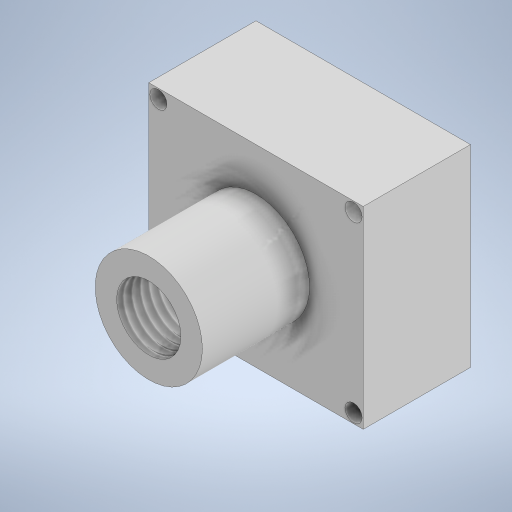
# Autodesk Inventor part: Practica 1 Sofia Lopez
Saved by Autodesk Inventor 2024 (Build 280153000, 153)
## iProperties
Created: 2024-02-06
Part Number: Practica 1 Sofia Lopez
Material: Generic
Document SubType Name: Sheet Metal
Designer: USUARIO
Density: 1 g/cm^3
Sheet Metal Rule: Default
Appearance: Default
Author: USUARIO
Autodesk Inventor part; units mm, degrees
ref_plane "YZ Plane" through (0, 0, 0) normal (1, 0, 0) x (0, 1, 0)
ref_plane "XZ Plane" through (0, 0, 0) normal (0, 1, 0) x (-1, 0, 0)
ref_plane "XY Plane" through (0, 0, 0) normal (0, 0, 1) x (1, 0, 0)
sketch "Sketch1" plane through (0, 0, 0) normal (0, 0, 1) x (1, 0, 0)
  line L0 (-50, 45) -> (50, 45)
  line L1 (50, 45) -> (50, -45)
  line L2 (50, -45) -> (-50, -45)
  line L3 (-50, -45) -> (-50, 45)
  line L4 (-50, 45) -> (50, -45) construction
  line L5 (50, 45) -> (-50, -45) construction
  point P0 (0, 0)
  constraints: 12 end point, 2 midpoint, 2 parallel, 1 horizontal, 1 perpendicular
extrude "Extrusion1" add sketch "Sketch1" against normal blind 50
sketch "Sketch2" plane through (0, 0, 0) normal (0, 0, 1) x (1, 0, 0)
  circle A0 centre (0, 0) radius 25
  constraints: 1 centre point, 1 coincident
extrude "Extrusion2" add sketch "Sketch2" along normal blind 50
sketch "Sketch3" plane through (0, 0, 50) normal (0, 0, 1) x (1, 0, 0)
  circle A0 centre (0, 0) radius 15
  constraints: 1 centre point, 1 coincident
extrude "Extrusion3" cut sketch "Sketch3" against normal blind 30
thread "Thread1" size "M50x4" class "6H" standard "ANSI Metric M Profile" full length
sketch "Sketch4" plane through (0, 0, 0) normal (0, 0, 1) x (1, 0, 0)
  line L0 (-50, 45) -> (50, 45) projected
  line L1 (-50, 45) -> (-41, 45)
  line L2 (-50, 36) -> (-50, 45)
  line L3 (50, 45) -> (41, 45)
  line L4 (50, 36) -> (50, 45)
  line L5 (50, -45.06) -> (41, -45.06)
  line L6 (50, -36.06) -> (50, -45.06)
  line L7 (-50, -45.06) -> (-41, -45.06)
  line L8 (-50, -36.06) -> (-50, -45.06)
  circle A0 centre (-45.5, 40.5) radius 4
  circle A1 centre (45.5, 40.5) radius 4
  circle A2 centre (45.5, -40.56) radius 4
  circle A3 centre (-45.5, -40.56) radius 4
  point P0 (0, 0)
  constraints: 16 end point, 4 centre point, 4 horizontal, 3 point on line
extrude "Extrusion4" cut sketch "Sketch4" against normal through all
equation "\"BendRadius\" = Thickness"
equation "\"BendReliefWidth\" = Thickness"
equation "\"BendReliefDepth\" = 0.5 * Thickness"
equation "\"CornerReliefSize\" = 4 * Thickness"
equation "\"MinimumRemnant\" = 2 * Thickness"
equation "\"TransitionRadius\" = BendRadius"
equation "\"JacobiRadiusSize\" = BendRadius"
equation "\"GapSize\" = Thickness"
equation "\"Thickness\" = 3.048"
body "Solid1"
